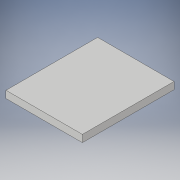
# Autodesk Inventor part: Screen Driver
Saved by Autodesk Inventor 2018 (Build 220112000, 112)
## iProperties
Created: 2017-05-31
Part Number: Screen Driver
Material: Generic
Document SubType Name: Modeling
Designer: Rishi
Density: 1 g/cm^3
Appearance: Default
Author: Rishi
Autodesk Inventor part; units mm, degrees
ref_plane "YZ Plane" through (0, 0, 0) normal (1, 0, 0) x (0, 1, 0)
ref_plane "XZ Plane" through (0, 0, 0) normal (0, 1, 0) x (-1, 0, 0)
ref_plane "XY Plane" through (0, 0, 0) normal (0, 0, 1) x (1, 0, 0)
sketch "Sketch1" plane through (0, 0, 0) normal (0, 1, 0) x (-1, 0, 0)
  line L0 (40.6, 48.7) -> (0, 48.7)
  line L1 (0, 48.7) -> (0, 0)
  line L2 (0, 0) -> (40.6, 0)
  line L3 (40.6, 0) -> (40.6, 48.7)
  dimension "d0" = 40.6
  dimension "d1" = 48.7
  constraints: 8 end point, 2 parallel, 1 horizontal, 1 perpendicular
  measures "d0" distance of L0.start L0.end
  measures "d1" distance of L2.end L0.start
extrude "Extrusion1" add sketch "Sketch1" along normal blind 3.8
body "Solid1"
